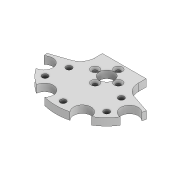
# Autodesk Inventor part: Cart wall
Saved by Autodesk Inventor 2020 (Build 240168000, 168)
## iProperties
Created: 2020-10-11
Part Number: Cart wall
Material: Generic
Document SubType Name: Modeling
Designer: ferrerx
Density: 1 g/cm^3
Appearance: Default
Author: ferrerx
Autodesk Inventor part; units mm, degrees
ref_plane "YZ Plane" through (0, 0, 0) normal (1, 0, 0) x (0, 1, 0)
ref_plane "XZ Plane" through (0, 0, 0) normal (0, 1, 0) x (-1, 0, 0)
ref_plane "XY Plane" through (0, 0, 0) normal (0, 0, 1) x (1, 0, 0)
sketch "Sketch1" plane through (0, 0, 0) normal (0, 1, 0) x (-1, 0, 0)
  line L0 (-22.552919, -44.014081) -> (22.447081, -44.014081)
  line L1 (-22.552919, -44.014081) -> (22.447081, -44.014081)
  line L2 (22.447081, 2.985919) -> (22.447081, -44.014081)
  line L3 (22.447081, 2.985919) -> (12.447081, 2.985919)
  line L4 (-22.552919, 2.985919) -> (-22.552919, -44.014081)
  line L5 (-22.552919, 2.985919) -> (-12.447081, 2.985919)
  arc A0 (-12.447081, 2.985919) -> (12.447081, 2.985919) centre (0, 4.13491) ccw
  circle A1 centre (-18.052919, -7.014081) radius 1.95
  circle A2 centre (-18.052919, -7.014081) radius 1.95
  circle A3 centre (17.947081, -7.014081) radius 1.95
  circle A4 centre (17.947081, -7.014081) radius 1.95
  circle A5 centre (0, -32.014081) radius 5.1
  circle A6 centre (-18.052919, -24.014168) radius 2
  circle A7 centre (-18, -40.014081) radius 2
  circle A8 centre (18, -40.014081) radius 2
  circle A9 centre (17.947081, -24.014168) radius 2
  line L6 (0, 4.13491) -> (0, -32.014081) construction
  point P0 (0, 0)
  dimension "d0" = 45
  dimension "d3" = 10
  dimension "d4" = 12.5
  dimension "d7" = 4.5
  dimension "d8" = 10
  dimension "d9" = 12
  dimension "d10" = 4
  dimension "d11" = 16
  dimension "d12" = 36
  dimension "d13" = 16
  dimension "d14" = 4.5
  dimension "d15" = 18
  dimension "d17" = 4.5
  dimension "d19" = 4
  dimension "d20" = 4
  dimension "d21" = 4
  dimension "d22" = 4
  dimension "d23" = 4
  dimension "d29" = 47
  dimension "d33" = 4.5
  dimension "d34" = 10
  constraints: 14 end point, 10 centre point, 3 coincident, 3 vertical, 2 collinear, 2 point on circle, 1 horizontal, 1 point on line
  measures "d0" distance of L0.start L0.end
  measures "d3" distance of L2.start L3.end
  measures "d4" radius of A0
  measures "d7" distance from line of L4 A1.centre
  measures "d8" distance from line of L5 A1.centre
  measures "d9" distance from line of L1 L6.end
  measures "d10" diameter of A7
  measures "d11" distance of A6.centre A7.centre
  measures "d12" distance of A8.centre A7.centre
  measures "d13" distance of A9.centre A8.centre
  measures "d14" distance from line of L2 A9.centre
  measures "d15" horizontal distance of A8.centre L6.end
  measures "d17" distance from line of L4 A6.centre
  measures "d19" diameter of A9
  measures "d20" diameter of A8
  measures "d21" diameter of A6
  measures "d22" distance from line of L0 A8.centre
  measures "d23" distance from line of L0 A7.centre
  measures "d29" distance between parallel lines of L0 L3
  measures "d33" distance from line of L2 A3.centre
  measures "d34" distance from line of L3 A3.centre
extrude "Extrusion1" add sketch "Sketch1" along normal blind 5
fillet "Fillet3" [suppressed]
fillet "Fillet4" [suppressed]
sketch "Sketch5" plane through (0, 5, 0) normal (0, 1, 0) x (1, 0, 0)
  arc A0 (12.447081, -2.985919) -> (-12.447081, -2.985919) centre (0, -4.13491) ccw
  arc A1 (12.447081, -2.985919) -> (-12.447081, -2.985919) centre (0, -4.13491) ccw
  line L0 (12.447081, -2.985919) -> (-12.447081, -2.985919)
  circle A2 centre (18.052919, 7.014081) radius 1.95
  circle A3 centre (18.052919, 7.014081) radius 1.95
  circle A4 centre (-17.947081, 7.014081) radius 1.95
  circle A5 centre (-17.947081, 7.014081) radius 1.95
  point P0 (0, 0)
  constraints: 3 centre point, 2 coincident, 2 end point, 2 point on circle, 1 concentric, 1 horizontal
extrude "Extrusion4" add sketch "Sketch5" against normal blind 5
sketch "Sketch8" plane through (0, 5, 0) normal (0, 1, 0) x (1, 0, 0)
  arc A0 (-25.305456, 28.046028) -> (25.305456, 28.046028) centre (0, 32) ccw
  arc A1 (-34.288263, 25.048052) -> (34.288263, 25.048052) centre (0, 32) ccw
  line L0 (-22.447081, -2.985919) -> (22.552919, -2.985919)
  line L1 (-22.447081, 44.014081) -> (-22.447081, -2.985919)
  line L2 (-22.447081, 29) -> (-34.288263, 25.048052)
  circle A2 centre (0, 32.014081) radius 5.1
  line L3 (0, 32.014081) -> (0, 0) construction
  line L4 (-22.447081, 29) -> (-22.447081, 19.665959)
  line L5 (34.288263, 25.048052) -> (22.552919, 29)
  line L6 (22.552919, -2.985919) -> (22.552919, 44.014081)
  line L7 (22.552919, 29) -> (22.552919, 19.860567)
  constraints: 10 end point, 6 point on circle, 5 point on line, 2 centre point, 1 coincident, 1 symmetric about line, 1 tangent, 1 vertical
extrude "Extrusion5" add sketch "Sketch8" against normal blind 5 contours L2 L1 A0 | A0 L1 A1 L2 | A0 L6 A1 L1 | L6 L5 A1
sketch "Sketch9" plane through (0, 5, 0) normal (0, 1, 0) x (1, 0, 0)
  circle A0 centre (0, 32) radius 34.985919
  line L0 (-22.447081, -2.985919) -> (22.552919, -2.985919)
  line L1 (22.552919, -2.985919) -> (22.552919, 5.253405)
  line L2 (22.552919, 5.253405) -> (22.552919, -2.985919)
  line L3 (22.552919, -2.985919) -> (-22.447081, -2.985919)
  line L4 (-22.447081, -2.985919) -> (-22.447081, 5.164518)
  point P0 (0, 0)
  point P1 (0, -2.985919)
  constraints: 6 end point, 2 collinear, 1 centre point, 1 point on circle, 1 tangent, 1 vertical
sketch "Sketch6" plane through (0, 5, 0) normal (0, 1, 0) x (1, 0, 0)
  circle A0 centre (0, 32.014081) radius 5.1
  circle A1 centre (0, 32.014081) radius 32.5 construction
  line L0 (0, 32.014081) -> (0, -0.485919) construction
  line L1 (0, 32.014081) -> (-13.735094, 2.559078) construction
  line L2 (0, 32.014081) -> (-29.455003, 18.278987) construction
  circle A2 centre (-13, 2.227339) radius 6
  circle A3 centre (-29.455003, 18.278987) radius 6
  circle A4 centre (13, 2.227339) radius 6
  circle A5 centre (29.455003, 18.278987) radius 6
  point P0 (0, 0)
  dimension "d49" = 65
  dimension "d50" = 12
  dimension "d51" = 12
  dimension "d52" = 25
  dimension "d53" = 40
  constraints: 6 end point, 5 centre point, 4 point on circle, 2 coincident, 2 symmetric about line, 1 vertical, 2 other
  measures "d49" diameter of A1
  measures "d50" diameter of A3
  measures "d51" diameter of A2
  measures "d52" angle of L1 L0
  measures "d53" angle of L1 L2
extrude "Extrusion6" cut sketch "Sketch9" against normal blind 5 contours A0 L0 L4 | L1 L0 A0
extrude "Extrusion7" cut sketch "Sketch6" against normal blind 5 contours A2 | A3 | A4 | A5
sketch "Sketch10" plane through (0, 5, 0) normal (0, 1, 0) x (1, 0, 0)
  circle A0 centre (0, 32.014081) radius 5.1
  circle A1 centre (0, 32.014081) radius 30 construction
  circle A2 centre (21.213203, 10.800877) radius 2
  circle A3 centre (0, 2.014081) radius 2
  circle A4 centre (-21.213203, 10.800877) radius 2
  line L0 (21.213203, 10.800877) -> (0, 32.014081) construction
  line L1 (0, 2.014081) -> (0, 32.014081) construction
  line L2 (-21.213203, 10.800877) -> (0, 32.014081) construction
  point P0 (0, 0)
  dimension "d60" = 60
  dimension "d61" = 4
  dimension "d62" = 4
  dimension "d63" = 4
  dimension "d64" = 45
  dimension "d65" = 45
  constraints: 6 end point, 4 centre point, 3 point on circle, 1 coincident, 1 vertical
  measures "d60" diameter of A1
  measures "d61" diameter of A2
  measures "d62" diameter of A3
  measures "d63" diameter of A4
  measures "d64" angle of L1 L2
  measures "d65" angle of L1 L0
extrude "Extrusion8" cut sketch "Sketch10" against normal blind 10 contours A2 | A3 | A4
sketch "Sketch11" plane through (0, 5, 0) normal (0, 1, 0) x (1, 0, 0)
  circle A0 centre (0, 32.014081) radius 5.1
  circle A1 centre (0, 32.014081) radius 8 construction
  circle A2 centre (0, 24.014081) radius 1.5
  point P0 (0, 0)
  dimension "d68" = 16
  dimension "d69" = 3
  constraints: 1 centre point, 1 coincident, 1 vertical alignment, 2 other
  measures "d69" diameter of A2
extrude "Extrusion9" cut sketch "Sketch11" against normal blind 10 contours A2
pattern_circular "Circular Pattern1" count 4 over 360 about axis through (0, 0, -32.014081) along (0, 1, 0) of "Extrusion9"
sketch "Sketch12" plane through (0, 5, 0) normal (0, 1, 0) x (1, 0, 0)
  line L0 (-22.447081, 44.014081) -> (-22.447081, 29)
  line L1 (-22.447081, 44.014081) -> (-14.947081, 44.014081)
  line L2 (-14.947081, 44.014081) -> (-14.947081, 29)
  line L3 (-14.947081, 29) -> (-22.447081, 29)
  line L4 (-22.447081, 29) -> (-22.447081, 44.014081)
  line L5 (22.552919, 29) -> (22.552919, 44.014081)
  line L6 (22.552919, 44.014081) -> (15.052919, 44.014081)
  line L7 (15.052919, 44.014081) -> (15.052919, 29)
  line L8 (15.052919, 29) -> (22.552919, 29)
  line L9 (22.552919, 29) -> (22.552919, 44.014081)
  point P0 (0, 0)
  dimension "d75" = 7.5
  dimension "d76" = 7.5
  constraints: 16 end point, 4 parallel, 2 horizontal, 2 perpendicular, 1 point on line
  measures "d75" distance of L5.end L6.end
  measures "d76" distance of L0.start L1.end
extrude "Extrusion10" cut sketch "Sketch12" against normal blind 10
fillet "Fillet6" radius 10 2 edges at (15.0529, 2.5, -29) (-14.9471, 2.5, -29)
thicken "Thicken1" operation add thickness 0.1 both sides no extend neighbours yes toward (0, 1, 0) faces at (9.884, 5, -17.948723)
chamfer "Chamfer1" distance 1.3 angle 45 4 edges at (8, 5.1, -30.5141) (-1.5, 5.1, -24.0141) (-8, 5.1, -33.5141) (1.5, 5.1, -40.0141)
body "Solid1"
